Autodesk Fusion 360 part; units mm, degrees
note: some values were not read from the file. Set by a fixed rule: which sketch regions a step uses.
(part 8 of 8)
sketch "Sketch6" plane through (0, 0, 0) normal (0, 0, 1) x (1, 0, 0)
  circle A0 centre (192.158, 102.8822) radius 3.75
  line L0 (-169.0689, -23.2426) -> (259.656, -23.2426)
  arc A1 (-174.0689, -18.2426) -> (-169.0689, -23.2426) centre (-169.0689, -18.2426) ccw
  line L1 (-174.0689, 118.4832) -> (-174.0689, -18.2426)
  arc A2 (-169.0689, 123.4832) -> (-174.0689, 118.4832) centre (-169.0689, 118.4832) ccw
  line L2 (259.656, 123.4832) -> (-169.0689, 123.4832)
  arc A3 (264.656, 118.4832) -> (259.656, 123.4832) centre (259.656, 118.4832) ccw
  line L3 (264.656, -18.2426) -> (264.656, 118.4832)
  arc A4 (259.656, -23.2426) -> (264.656, -18.2426) centre (259.656, -18.2426) ccw
  line L4 (114.998, 83.109) -> (114.998, -11.1417)
  arc A5 (114.998, 83.109) -> (113.998, 84.109) centre (113.998, 83.109) ccw
  line L5 (-168.37, 84.109) -> (113.998, 84.109)
  arc A6 (-168.37, 84.109) -> (-169.37, 83.109) centre (-168.37, 83.109) ccw
  line L6 (-169.37, -11.1417) -> (-169.37, 83.109)
  arc A7 (-169.37, -11.1417) -> (-168.37, -12.1417) centre (-168.37, -11.1417) ccw
  line L7 (113.998, -12.1417) -> (-168.37, -12.1417)
  arc A8 (113.998, -12.1417) -> (114.998, -11.1417) centre (113.998, -11.1417) ccw
  line L8 (-150.3191, 92.6332) -> (-168.37, 92.6332)
  arc A9 (-150.3191, 92.6332) -> (-149.3191, 93.6332) centre (-150.3191, 93.6332) ccw
  line L9 (-149.3191, 111.6852) -> (-149.3191, 93.6332)
  arc A10 (-149.3191, 111.6852) -> (-150.3191, 112.6852) centre (-150.3191, 111.6852) ccw
  line L10 (-168.37, 112.6852) -> (-150.3191, 112.6852)
  arc A11 (-168.37, 112.6852) -> (-169.37, 111.6852) centre (-168.37, 111.6852) ccw
  line L11 (-169.37, 93.6332) -> (-169.37, 111.6852)
  arc A12 (-169.37, 93.6332) -> (-168.37, 92.6332) centre (-168.37, 93.6332) ccw
  line L12 (121.142, 93.6332) -> (121.142, 111.6852)
  arc A13 (121.142, 93.6332) -> (122.142, 92.6332) centre (122.142, 93.6332) ccw
  line L13 (178.292, 92.6332) -> (122.142, 92.6332)
  arc A14 (178.292, 92.6332) -> (179.292, 93.6332) centre (178.292, 93.6332) ccw
  line L14 (179.292, 111.6852) -> (179.292, 93.6332)
  arc A15 (179.292, 111.6852) -> (178.292, 112.6852) centre (178.292, 111.6852) ccw
  line L15 (122.142, 112.6852) -> (178.292, 112.6852)
  arc A16 (122.142, 112.6852) -> (121.142, 111.6852) centre (122.142, 111.6852) ccw
  line L16 (179.292, 83.109) -> (179.292, 46.0083)
  arc A17 (179.292, 83.109) -> (178.292, 84.109) centre (178.292, 83.109) ccw
  line L17 (122.142, 84.109) -> (178.292, 84.109)
  arc A18 (122.142, 84.109) -> (121.142, 83.109) centre (122.142, 83.109) ccw
  line L18 (121.142, 46.0083) -> (121.142, 83.109)
  arc A19 (121.142, -11.1417) -> (122.142, -12.1417) centre (122.142, -11.1417) ccw
  line L19 (178.292, -12.1417) -> (122.142, -12.1417)
  arc A20 (178.292, -12.1417) -> (179.292, -11.1417) centre (178.292, -11.1417) ccw
  line L20 (-131.2701, 93.6332) -> (-131.2701, 111.6852)
  arc A21 (-131.2701, 93.6332) -> (-130.2701, 92.6332) centre (-130.2701, 93.6332) ccw
  line L21 (-55.069, 92.6332) -> (-130.2701, 92.6332)
  arc A22 (-55.069, 92.6332) -> (-54.069, 93.6332) centre (-55.069, 93.6332) ccw
  line L22 (-54.069, 111.6852) -> (-54.069, 93.6332)
  arc A23 (-54.069, 111.6852) -> (-55.069, 112.6852) centre (-55.069, 111.6852) ccw
  line L23 (-130.2701, 112.6852) -> (-55.069, 112.6852)
  arc A24 (-130.2701, 112.6852) -> (-131.2701, 111.6852) centre (-130.2701, 111.6852) ccw
  line L24 (40.18, 93.6332) -> (40.18, 111.6852)
  arc A25 (40.18, 93.6332) -> (41.18, 92.6332) centre (41.18, 93.6332) ccw
  line L25 (116.381, 92.6332) -> (41.18, 92.6332)
  arc A26 (116.381, 92.6332) -> (117.381, 93.6332) centre (116.381, 93.6332) ccw
  line L26 (117.381, 111.6852) -> (117.381, 93.6332)
  arc A27 (117.381, 111.6852) -> (116.381, 112.6852) centre (116.381, 111.6852) ccw
  line L27 (41.18, 112.6852) -> (116.381, 112.6852)
  arc A28 (41.18, 112.6852) -> (40.18, 111.6852) centre (41.18, 111.6852) ccw
  line L28 (184.055, 84.109) -> (259.257, 84.109)
  arc A29 (184.055, 84.109) -> (183.055, 83.109) centre (184.055, 83.109) ccw
  line L29 (183.055, -11.1417) -> (183.055, 83.109)
  arc A30 (183.055, -11.1417) -> (184.055, -12.1417) centre (184.055, -11.1417) ccw
  line L30 (259.257, -12.1417) -> (184.055, -12.1417)
  arc A31 (259.257, -12.1417) -> (260.257, -11.1417) centre (259.257, -11.1417) ccw
  line L31 (260.257, 83.109) -> (260.257, -11.1417)
  arc A32 (260.257, 83.109) -> (259.257, 84.109) centre (259.257, 83.109) ccw
  line L32 (-45.545, 93.6332) -> (-45.545, 111.6852)
  arc A33 (-45.545, 93.6332) -> (-44.545, 92.6332) centre (-44.545, 93.6332) ccw
  line L33 (30.656, 92.6332) -> (-44.545, 92.6332)
  arc A34 (30.656, 92.6332) -> (31.656, 93.6332) centre (30.656, 93.6332) ccw
  line L34 (31.656, 111.6852) -> (31.656, 93.6332)
  arc A35 (31.656, 111.6852) -> (30.656, 112.6852) centre (30.656, 111.6852) ccw
  line L35 (-44.545, 112.6852) -> (30.656, 112.6852)
  arc A36 (-44.545, 112.6852) -> (-45.545, 111.6852) centre (-44.545, 111.6852) ccw
  arc A37 (121.142, 46.0083) -> (122.142, 45.0083) centre (122.142, 46.0083) ccw
  line L36 (178.292, 45.0083) -> (122.142, 45.0083)
  arc A38 (178.292, 45.0083) -> (179.292, 46.0083) centre (178.292, 46.0083) ccw
  line L37 (141.192, 26.959) -> (159.242, 26.959)
  arc A39 (141.192, 26.959) -> (140.192, 25.959) centre (141.192, 25.959) ccw
  line L38 (140.192, 8.9091) -> (140.192, 25.959)
  arc A40 (139.192, 7.9091) -> (140.192, 8.9091) centre (139.192, 8.9091) ccw
  line L39 (122.142, 7.9091) -> (139.192, 7.9091)
  arc A41 (122.142, 7.9091) -> (121.142, 6.9091) centre (122.142, 6.9091) ccw
  line L40 (121.142, -11.1417) -> (121.142, 6.9091)
  line L41 (179.292, 6.9091) -> (179.292, -11.1417)
  arc A42 (179.292, 6.9091) -> (178.292, 7.9091) centre (178.292, 6.9091) ccw
  line L42 (161.242, 7.9091) -> (178.292, 7.9091)
  arc A43 (160.242, 8.9091) -> (161.242, 7.9091) centre (161.242, 8.9091) ccw
  line L43 (160.242, 25.959) -> (160.242, 8.9091)
  arc A44 (160.242, 25.959) -> (159.242, 26.959) centre (159.242, 25.959) ccw
  line L44 (-152.2251, 143.5079) -> (-92.1638, -45.4351)
  line L45 (-148.4131, 144.7197) -> (-88.3518, -44.2233)
  line L46 (-92.1638, -45.4351) -> (-88.3518, -44.2233)
  line L47 (-152.2251, 143.5079) -> (-148.4131, 144.7197)
  line L48 (-138.4131, 144.7197) -> (-78.3518, -44.2233)
  line L49 (-142.2251, 143.5079) -> (-82.1638, -45.4351)
  line L50 (-142.2251, 143.5079) -> (-138.4131, 144.7197)
  line L51 (-82.1638, -45.4351) -> (-78.3518, -44.2233)
  line L52 (-128.4131, 144.7197) -> (-68.3518, -44.2233)
  line L53 (-132.2251, 143.5079) -> (-72.1638, -45.4351)
  line L54 (-132.2251, 143.5079) -> (-128.4131, 144.7197)
  line L55 (-72.1638, -45.4351) -> (-68.3518, -44.2233)
  line L56 (-118.4131, 144.7197) -> (-58.3518, -44.2233)
  line L57 (-122.2251, 143.5079) -> (-62.1638, -45.4351)
  line L58 (-122.2251, 143.5079) -> (-118.4131, 144.7197)
  line L59 (-62.1638, -45.4351) -> (-58.3518, -44.2233)
  line L60 (-108.4131, 144.7197) -> (-48.3518, -44.2233)
  line L61 (-112.2251, 143.5079) -> (-52.1638, -45.4351)
  line L62 (-112.2251, 143.5079) -> (-108.4131, 144.7197)
  line L63 (-52.1638, -45.4351) -> (-48.3518, -44.2233)
  line L64 (-98.4131, 144.7197) -> (-38.3518, -44.2233)
  line L65 (-102.2251, 143.5079) -> (-42.1638, -45.4351)
  line L66 (-102.2251, 143.5079) -> (-98.4131, 144.7197)
  line L67 (-42.1638, -45.4351) -> (-38.3518, -44.2233)
  line L68 (-88.4131, 144.7197) -> (-28.3518, -44.2233)
  line L69 (-92.2251, 143.5079) -> (-32.1638, -45.4351)
  line L70 (-92.2251, 143.5079) -> (-88.4131, 144.7197)
  line L71 (-32.1638, -45.4351) -> (-28.3518, -44.2233)
  line L72 (-78.4131, 144.7197) -> (-18.3518, -44.2233)
  line L73 (-82.2251, 143.5079) -> (-22.1638, -45.4351)
  line L74 (-82.2251, 143.5079) -> (-78.4131, 144.7197)
  line L75 (-22.1638, -45.4351) -> (-18.3518, -44.2233)
  line L76 (-68.4131, 144.7197) -> (-8.3518, -44.2233)
  line L77 (-72.2251, 143.5079) -> (-12.1638, -45.4351)
  line L78 (-72.2251, 143.5079) -> (-68.4131, 144.7197)
  line L79 (-12.1638, -45.4351) -> (-8.3518, -44.2233)
  line L80 (-58.4131, 144.7197) -> (1.6482, -44.2233)
  line L81 (-62.2251, 143.5079) -> (-2.1638, -45.4351)
  line L82 (-62.2251, 143.5079) -> (-58.4131, 144.7197)
  line L83 (-2.1638, -45.4351) -> (1.6482, -44.2233)
  line L84 (-48.4131, 144.7197) -> (11.6482, -44.2233)
  line L85 (-52.2251, 143.5079) -> (7.8362, -45.4351)
  line L86 (-52.2251, 143.5079) -> (-48.4131, 144.7197)
  line L87 (7.8362, -45.4351) -> (11.6482, -44.2233)
  line L88 (-38.4131, 144.7197) -> (21.6482, -44.2233)
  line L89 (-42.2251, 143.5079) -> (17.8362, -45.4351)
  line L90 (-42.2251, 143.5079) -> (-38.4131, 144.7197)
  line L91 (17.8362, -45.4351) -> (21.6482, -44.2233)
  line L92 (-28.4131, 144.7197) -> (31.6482, -44.2233)
  line L93 (-32.2251, 143.5079) -> (27.8362, -45.4351)
  line L94 (-32.2251, 143.5079) -> (-28.4131, 144.7197)
  line L95 (27.8362, -45.4351) -> (31.6482, -44.2233)
  line L96 (-18.4131, 144.7197) -> (41.6482, -44.2233)
  line L97 (-22.2251, 143.5079) -> (37.8362, -45.4351)
  line L98 (-22.2251, 143.5079) -> (-18.4131, 144.7197)
  line L99 (37.8362, -45.4351) -> (41.6482, -44.2233)
  line L100 (-8.4131, 144.7197) -> (51.6482, -44.2233)
  line L101 (-12.2251, 143.5079) -> (47.8362, -45.4351)
  line L102 (-12.2251, 143.5079) -> (-8.4131, 144.7197)
  line L103 (47.8362, -45.4351) -> (51.6482, -44.2233)
  line L104 (1.5869, 144.7197) -> (61.6482, -44.2233)
  line L105 (-2.2251, 143.5079) -> (57.8362, -45.4351)
  line L106 (-2.2251, 143.5079) -> (1.5869, 144.7197)
  line L107 (57.8362, -45.4351) -> (61.6482, -44.2233)
  line L108 (11.5869, 144.7197) -> (71.6482, -44.2233)
  line L109 (7.7749, 143.5079) -> (67.8362, -45.4351)
  line L110 (7.7749, 143.5079) -> (11.5869, 144.7197)
  line L111 (67.8362, -45.4351) -> (71.6482, -44.2233)
  line L112 (21.5869, 144.7197) -> (81.6482, -44.2233)
  line L113 (17.7749, 143.5079) -> (77.8362, -45.4351)
  line L114 (17.7749, 143.5079) -> (21.5869, 144.7197)
  line L115 (77.8362, -45.4351) -> (81.6482, -44.2233)
  line L116 (31.5869, 144.7197) -> (91.6482, -44.2233)
  line L117 (27.7749, 143.5079) -> (87.8362, -45.4351)
  line L118 (27.7749, 143.5079) -> (31.5869, 144.7197)
  line L119 (87.8362, -45.4351) -> (91.6482, -44.2233)
  line L120 (31.5869, 144.7197) -> (91.6482, -44.2233)
  line L121 (27.7749, 143.5079) -> (87.8362, -45.4351)
  line L122 (27.7749, 143.5079) -> (31.5869, 144.7197)
  line L123 (87.8362, -45.4351) -> (91.6482, -44.2233)
  line L124 (41.5869, 144.7197) -> (101.6482, -44.2233)
  line L125 (37.7749, 143.5079) -> (97.8362, -45.4351)
  line L126 (37.7749, 143.5079) -> (41.5869, 144.7197)
  line L127 (97.8362, -45.4351) -> (101.6482, -44.2233)
  line L128 (51.5869, 144.7197) -> (111.6482, -44.2233)
  line L129 (47.7749, 143.5079) -> (107.8362, -45.4351)
  line L130 (47.7749, 143.5079) -> (51.5869, 144.7197)
  line L131 (107.8362, -45.4351) -> (111.6482, -44.2233)
  line L132 (61.5869, 144.7197) -> (121.6482, -44.2233)
  line L133 (57.7749, 143.5079) -> (117.8362, -45.4351)
  line L134 (57.7749, 143.5079) -> (61.5869, 144.7197)
  line L135 (117.8362, -45.4351) -> (121.6482, -44.2233)
  line L136 (71.5869, 144.7197) -> (131.6482, -44.2233)
  line L137 (67.7749, 143.5079) -> (127.8362, -45.4351)
  line L138 (67.7749, 143.5079) -> (71.5869, 144.7197)
  line L139 (127.8362, -45.4351) -> (131.6482, -44.2233)
  line L140 (81.5869, 144.7197) -> (141.6482, -44.2233)
  line L141 (77.7749, 143.5079) -> (137.8362, -45.4351)
  line L142 (77.7749, 143.5079) -> (81.5869, 144.7197)
  line L143 (137.8362, -45.4351) -> (141.6482, -44.2233)
  line L144 (91.5869, 144.7197) -> (151.6482, -44.2233)
  line L145 (87.7749, 143.5079) -> (147.8362, -45.4351)
  line L146 (87.7749, 143.5079) -> (91.5869, 144.7197)
  line L147 (147.8362, -45.4351) -> (151.6482, -44.2233)
  line L148 (101.5869, 144.7197) -> (161.6482, -44.2233)
  line L149 (97.7749, 143.5079) -> (157.8362, -45.4351)
  line L150 (97.7749, 143.5079) -> (101.5869, 144.7197)
  line L151 (157.8362, -45.4351) -> (161.6482, -44.2233)
  line L152 (111.5869, 144.7197) -> (171.6482, -44.2233)
  line L153 (107.7749, 143.5079) -> (167.8362, -45.4351)
  line L154 (107.7749, 143.5079) -> (111.5869, 144.7197)
  line L155 (167.8362, -45.4351) -> (171.6482, -44.2233)
  line L156 (121.5869, 144.7197) -> (181.6482, -44.2233)
  line L157 (117.7749, 143.5079) -> (177.8362, -45.4351)
  line L158 (117.7749, 143.5079) -> (121.5869, 144.7197)
  line L159 (177.8362, -45.4351) -> (181.6482, -44.2233)
  line L160 (131.5869, 144.7197) -> (191.6482, -44.2233)
  line L161 (127.7749, 143.5079) -> (187.8362, -45.4351)
  line L162 (127.7749, 143.5079) -> (131.5869, 144.7197)
  line L163 (187.8362, -45.4351) -> (191.6482, -44.2233)
  line L164 (141.5869, 144.7197) -> (201.6482, -44.2233)
  line L165 (137.7749, 143.5079) -> (197.8362, -45.4351)
  line L166 (137.7749, 143.5079) -> (141.5869, 144.7197)
  line L167 (197.8362, -45.4351) -> (201.6482, -44.2233)
  line L168 (151.5869, 144.7197) -> (211.6482, -44.2233)
  line L169 (147.7749, 143.5079) -> (207.8362, -45.4351)
  line L170 (147.7749, 143.5079) -> (151.5869, 144.7197)
  line L171 (207.8362, -45.4351) -> (211.6482, -44.2233)
  line L172 (161.5869, 144.7197) -> (221.6482, -44.2233)
  line L173 (157.7749, 143.5079) -> (217.8362, -45.4351)
  line L174 (157.7749, 143.5079) -> (161.5869, 144.7197)
  line L175 (217.8362, -45.4351) -> (221.6482, -44.2233)
  line L176 (-158.4131, 144.7197) -> (-98.3518, -44.2233)
  line L177 (-162.2251, 143.5079) -> (-102.1638, -45.4351)
  line L178 (-162.2251, 143.5079) -> (-158.4131, 144.7197)
  line L179 (-102.1638, -45.4351) -> (-98.3518, -44.2233)
  line L180 (-168.4131, 144.7197) -> (-108.3518, -44.2233)
  line L181 (-172.2251, 143.5079) -> (-112.1638, -45.4351)
  line L182 (-172.2251, 143.5079) -> (-168.4131, 144.7197)
  line L183 (-112.1638, -45.4351) -> (-108.3518, -44.2233)
  line L184 (-178.4131, 144.7197) -> (-118.3518, -44.2233)
  line L185 (-182.2251, 143.5079) -> (-122.1638, -45.4351)
  line L186 (-182.2251, 143.5079) -> (-178.4131, 144.7197)
  line L187 (-122.1638, -45.4351) -> (-118.3518, -44.2233)
  line L188 (-188.4131, 144.7197) -> (-128.3518, -44.2233)
  line L189 (-192.2251, 143.5079) -> (-132.1638, -45.4351)
  line L190 (-192.2251, 143.5079) -> (-188.4131, 144.7197)
  line L191 (-132.1638, -45.4351) -> (-128.3518, -44.2233)
  line L192 (-198.4131, 144.7197) -> (-138.3518, -44.2233)
  line L193 (-202.2251, 143.5079) -> (-142.1638, -45.4351)
  line L194 (-202.2251, 143.5079) -> (-198.4131, 144.7197)
  line L195 (-142.1638, -45.4351) -> (-138.3518, -44.2233)
  line L196 (-208.4131, 144.7197) -> (-148.3518, -44.2233)
  line L197 (-212.2251, 143.5079) -> (-152.1638, -45.4351)
  line L198 (-212.2251, 143.5079) -> (-208.4131, 144.7197)
  line L199 (-152.1638, -45.4351) -> (-148.3518, -44.2233)
  line L200 (-218.4131, 144.7197) -> (-158.3518, -44.2233)
  line L201 (-222.2251, 143.5079) -> (-162.1638, -45.4351)
  line L202 (-222.2251, 143.5079) -> (-218.4131, 144.7197)
  line L203 (-162.1638, -45.4351) -> (-158.3518, -44.2233)
  constraint perpendicular L45 L46
  constraint perpendicular L45 L47
  constraint perpendicular L48 L51
  constraint perpendicular L48 L50
  constraint perpendicular L52 L55
  constraint perpendicular L52 L54
  constraint perpendicular L56 L59
  constraint perpendicular L56 L58
  constraint perpendicular L60 L63
  constraint perpendicular L60 L62
  constraint perpendicular L64 L67
  constraint perpendicular L64 L66
  constraint perpendicular L68 L71
  constraint perpendicular L68 L70
  constraint perpendicular L72 L75
  constraint perpendicular L72 L74
  constraint perpendicular L76 L79
  constraint perpendicular L76 L78
  constraint perpendicular L80 L83
  constraint perpendicular L80 L82
  constraint perpendicular L84 L87
  constraint perpendicular L84 L86
  constraint perpendicular L88 L91
  constraint perpendicular L88 L90
  constraint perpendicular L92 L95
  constraint perpendicular L92 L94
  constraint perpendicular L96 L99
  constraint perpendicular L96 L98
  constraint perpendicular L100 L103
  constraint perpendicular L100 L102
  constraint perpendicular L104 L107
  constraint perpendicular L104 L106
  constraint perpendicular L108 L111
  constraint perpendicular L108 L110
  constraint perpendicular L112 L115
  constraint perpendicular L112 L114
  constraint perpendicular L116 L119
  constraint perpendicular L116 L118
  constraint perpendicular L120 L123
  constraint perpendicular L120 L122
  constraint perpendicular L124 L127
  constraint perpendicular L124 L126
  constraint perpendicular L128 L131
  constraint perpendicular L128 L130
  constraint perpendicular L132 L135
  constraint perpendicular L132 L134
  constraint perpendicular L136 L139
  constraint perpendicular L136 L138
  constraint perpendicular L140 L143
  constraint perpendicular L140 L142
  constraint perpendicular L144 L147
  constraint perpendicular L144 L146
  constraint perpendicular L148 L151
  constraint perpendicular L148 L150
  constraint perpendicular L152 L155
  constraint perpendicular L152 L154
  constraint perpendicular L156 L159
  constraint perpendicular L156 L158
  constraint perpendicular L160 L163
  constraint perpendicular L160 L162
  constraint perpendicular L164 L167
  constraint perpendicular L164 L166
  constraint perpendicular L168 L171
  constraint perpendicular L168 L170
  constraint perpendicular L172 L175
  constraint perpendicular L172 L174
  constraint perpendicular L176 L179
  constraint perpendicular L176 L178
  constraint perpendicular L180 L183
  constraint perpendicular L180 L182
  constraint perpendicular L184 L187
  constraint perpendicular L184 L186
  constraint perpendicular L188 L191
  constraint perpendicular L188 L190
  constraint perpendicular L192 L195
  constraint perpendicular L192 L194
  constraint perpendicular L196 L199
  constraint perpendicular L196 L198
  constraint perpendicular L200 L203
  constraint perpendicular L200 L202
extrude "Extrude8" add sketch "Sketch6" along normal blind 0.5 from surface at 7.5 contours L0 A7 L7 L197 L200 | L0 L7 L196 L197 | L1 L6 L197 L200 | L1 L6 L196 L197 | L0 L7 L189 L192 | L0 L7 L188 L189 | L1 L6 L189 L192 | L1 A6 L6 L188 L189 | L0 L7 L181 L184 | L0 L7 L180 L181 | L5 L8 L181 L184 | L5 L8 L180 L181 | A2 L2 L10 L181 L184 | L0 L7 L44 L176 | L0 L7 L44 L45 | L2 L10 L180 L181 | L2 L5 L44 L176 | L2 L5 L44 L45 | L0 L7 L48 L53 | L0 L7 L52 L53 | L5 L21 L48 L53 | L5 L21 L52 L53 | L2 L23 L48 L53 | L0 L7 L56 L61 | L2 L23 L52 L53 | L0 L7 L60 L61 | L5 L21 L56 L61 | L5 L21 L60 L61 | L2 L23 L56 L61 | L0 L7 L64 L69 | L2 L23 L60 L61 | L0 L7 L68 L69 | L5 L21 L64 L69 | L5 L21 L68 L69 | L2 L23 L64 L69 | L0 L7 L72 L77 | L2 L23 L68 L69 | L0 L7 L76 L77 | L5 L21 L72 L77 | L5 L21 A22 L22 L76 L77 | L2 L23 L72 L77 | L0 L7 L80 L85 | L2 L23 L76 L77 | L0 L7 L84 L85 | L5 L33 L80 L85 | L5 L33 L84 L85 | L2 L32 L35 A36 L80 L85 | L0 L7 L88 L93 | L2 L35 L84 L85 | L0 L7 L92 L93 | L5 L33 L88 L93 | L5 L33 L92 L93 | L2 L35 L88 L93 | L0 L7 L96 L101 | L2 L35 L92 L93 | L0 L7 L100 L101 | L5 L33 L96 L101 | L5 L33 L100 L101 | L2 L35 L96 L101 | L0 L7 L104 L109 | L2 L35 L100 L101 | L0 L7 L108 L109 | L5 L33 L104 L109 | L5 L33 L108 L109 | L2 L35 L104 L109 | L0 L7 L112 L117 L121 | L2 L35 L108 L109 | L0 L7 L116 L117 L120 L121 | L2 L5 L24 A25 L25 L112 L117 L121 | L5 L25 L116 L117 L120 L121 | L0 L7 L124 L129 | L2 L24 L27 A28 L116 L117 L120 L121 | L0 L7 L128 L129 | L5 L25 L124 L129 | L5 L25 L128 L129 | L2 L27 L124 L129 | L0 L4 L7 A8 L132 L137 | L2 L27 L128 L129 | L0 L4 A19 L136 L137 | L5 L25 L132 L137 | L5 L25 L136 L137 | L2 L27 L132 L137 | L0 L19 L140 L145 | L2 L27 L136 L137 | L0 L19 L144 L145 | L4 L39 L140 L145 | L4 L18 A37 L36 L39 L144 L145 | L5 L25 L140 L145 | L5 L25 L144 L145 | L2 L27 L140 L145 | L0 L19 L148 L153 | L2 L27 L144 L145 | L0 L19 L152 L153 | L36 L37 A39 L38 L148 L153 | L36 L37 L152 L153 | L2 L12 A13 L13 L17 A18 L26 A27 L27 L148 L153 | L0 L19 L156 L161 | L2 L12 A16 L152 L153 | L0 L19 A20 L41 L160 L161 | L13 L17 L152 L153 | L36 L37 L42 L43 A44 L156 L161 | L36 L42 L160 L161 | L2 L15 L156 L161 | L0 L30 L164 L169 | L13 L17 L156 L161 | L2 L15 L160 L161 | L0 L30 L168 L169 | L13 L17 L160 L161 | L29 L36 A38 L164 L169 | L16 L29 A38 L168 L169 | L2 L15 L164 L169 | L13 L17 L164 L169 | L2 L15 L168 L169 | L13 L17 L168 L169 bodies 3
sketch "Sketch7" plane through (0, 0, 0) normal (1, 0, 0) x (0, 1, 0)
  line L0 (-18.2426, 0) -> (-23.2426, 0)
  line L1 (118.4832, 0) -> (-18.2426, 0)
  line L2 (123.4832, 0) -> (118.4832, 0)
  line L3 (-23.2426, 0) -> (-23.2426, 7.5)
  line L4 (123.4832, 0) -> (123.4832, 8)
  line L5 (-23.2426, 0) -> (-16.1638, 8.4362)
  line L6 (-23.2426, 0) -> (-12.2299, 0) construction
  line L7 (39.6139, 8) -> (36.6786, 8)
  line L8 (53.3549, 8) -> (39.6139, 8)
  line L9 (68.137, 8) -> (53.3549, 8)
  line L10 (99.5953, 8) -> (68.137, 8)
  line L11 (122.8703, 8) -> (112.6852, 8)
  line L12 (123.4832, 8) -> (122.8703, 8)
  line L13 (-23.2426, 7.5) -> (-23.2426, 8)
  line L14 (-12.1244, 8) -> (-23.2426, 8)
  line L15 (-9.5618, 8) -> (-11.1417, 8)
  line L16 (-11.1417, 8) -> (-12.1244, 8)
  line L17 (5.2203, 8) -> (-9.5618, 8)
  line L18 (36.6786, 8) -> (5.2203, 8)
  line L19 (112.6852, 8) -> (99.5953, 8)
  dimension "d251" = 50
  constraint horizontal L6
  constraint coincident L0.end L3.start
  measures "d251" angle of L5 L6
extrude "Extrude6" cut sketch "Sketch4" against normal blind 1 from surface at 7.5 bodies 3
